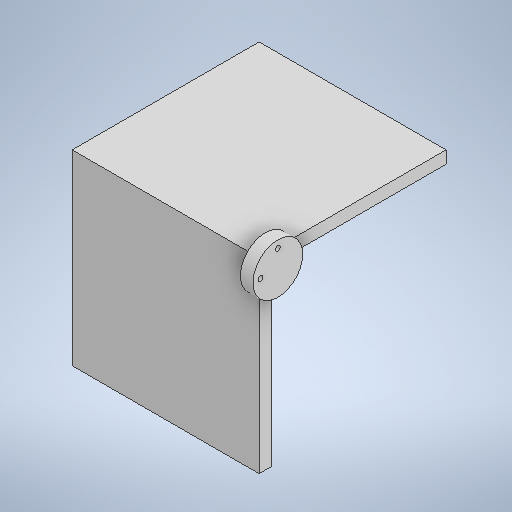
# Autodesk Inventor part: 排出機構
Saved by Autodesk Inventor 2026.2 (Build 302298010, 298A)
## iProperties
Created: 2026-05-18
Part Number: 排出機構
Material: 一般
Document SubType Name: Modeling
Designer: Yagis
Density: 1 g/cm^3
Appearance: 既定
Author: Yagis
Autodesk Inventor part; units mm, degrees
ref_plane "YZ Plane" through (0, 0, 0) normal (1, 0, 0) x (0, 1, 0)
ref_plane "XZ Plane" through (0, 0, 0) normal (0, 1, 0) x (-1, 0, 0)
ref_plane "XY Plane" through (0, 0, 0) normal (0, 0, 1) x (1, 0, 0)
sketch "スケッチ2" plane through (0, 0, 0) normal (1, 0, 0) x (0, 1, 0)
  line L0 (0, 0) -> (5, 0)
  line L1 (5, 0) -> (5, -75)
  line L2 (5, -75) -> (0, -75)
  line L3 (0, -75) -> (0, 0)
  line L4 (0, 0) -> (-70, 0)
  line L5 (-70, 0) -> (-70, -5)
  line L6 (-70, -5) -> (0, -5)
  line L7 (0, -5) -> (0, 0)
  point P0 (-70, -2.5)
  point P1 (0, -5)
  dimension "d0" = 75
  dimension "d1" = 75
  dimension "d2" = 5
  dimension "d3" = 5
  constraints: 16 end point, 4 parallel, 2 horizontal, 2 perpendicular, 1 midpoint
  measures "d0" distance of L0.end L1.end
  measures "d1" distance from line of point (-70, -2.5) L1
  measures "d2" distance of L1.end L2.end
  measures "d3" distance of L4.end L5.end
extrude "押し出し1" add sketch "スケッチ2" along normal blind 75
sketch "スケッチ4" plane through (75, 0, 0) normal (1, 0, 0) x (0, 0, -1)
  line L0 (0, 0) -> (13, 0)
  line L1 (0, 0) -> (5, 0)
  line L2 (75, 5) -> (0, 5) projected
  line L3 (0, 5) -> (0, -70) projected
  circle A0 centre (2.5, 2.5) radius 10
  dimension "d32" = 2.5
  dimension "d33" = 2.5
  dimension "d34" = 20
  constraints: 4 end point, 2 horizontal, 1 centre point, 1 coincident
  measures "d32" distance from line of point (2.5, 2.5) L2
  measures "d33" distance from line of L3 point (2.5, 2.5)
  measures "d34" diameter of A0
extrude "押し出し2" add sketch "スケッチ4" along normal blind 5
sketch "スケッチ7" plane through (80, 2.5, -2.5) normal (1, 0, 0) x (0, 0, -1)
  point P0 (-2.5, -2.5)
  point P1 (0, 7)
  point P2 (-7, 0)
  point P3 (0, 0)
  dimension "d35" = 7
  dimension "d36" = 7
  constraints: 1 horizontal alignment, 1 vertical alignment, 1 other
  measures "d35" distance of point (0, 7) point (0, 0)
  measures "d36" distance of point (0, 0) point (-7, 0)
hole "穴2" at (80, 9.5, -2.5) at (80, 2.5, 4.5) direction (-1, 0, 0) diameter 2 depth 8.1 tip angle 118
